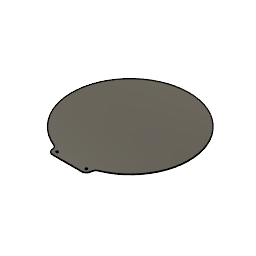
Delta Build Sheet (Autodesk Fusion 360 design; units mm, degrees)
part number: 180mm Square Bed
Autodesk Fusion 360 part; units mm, degrees
sketch "Round Bed" plane through (0, 0, 0) normal (0, 0, 1) x (1, 0, 0)
  line L0 (-90.1561, -90.1561) -> (90.1561, -90.1561) construction
  line L1 (90.1561, -90.1561) -> (90.1561, 90.1561) construction
  line L2 (90.1561, 90.1561) -> (-90.1561, 90.1561) construction
  line L3 (-90.1561, 90.1561) -> (-90.1561, -90.1561) construction
  line L4 (-90.1561, -90.1561) -> (90.1561, 90.1561) construction
  line L5 (90.1561, -90.1561) -> (-90.1561, 90.1561) construction
  line L6 (-31.875, -137.5) -> (31.875, -137.5)
  line L7 (0, 0) -> (0, -137.5) construction
  arc A0 (-42.0024, -127.3726) -> (-31.875, -137.5) centre (-31.875, -127.3726) ccw
  arc A1 (-42.0024, -127.3726) -> (-48.2938, -117.9998) centre (-52.1298, -127.3726) ccw
  arc A2 (31.875, -137.5) -> (42.0024, -127.3726) centre (31.875, -127.3726) ccw
  arc A3 (48.2938, -117.9998) -> (42.0024, -127.3726) centre (52.1298, -127.3726) ccw
  circle A4 centre (-31.875, -127.3726) radius 2
  circle A5 centre (31.875, -127.3726) radius 2
  arc A6 (48.2938, -117.9998) -> (-48.2938, -117.9998) centre (0, 0) ccw
  dimension "d4" = 255
  dimension "d6" = 63.75
  dimension "d7" = 137.5
  dimension "d10" = 4
  constraint coincident L7.start A6.centre
  constraint horizontal L0
  constraint perpendicular L0 L1
  constraint parallel L0 L2
  constraint parallel L1 L3
  constraint coincident L4 L7.start
  constraint coincident L5 L7.start
  constraint coincident L0.start A6
  constraint coincident L0.end A6
  constraint equal L2 L3
  constraint horizontal L6
  constraint midpoint L6 L7.end
  constraint vertical L7
  constraint tangent L6 A0
  constraint tangent A1 A6
  constraint tangent L6 A2
  constraint tangent A3 A6
  constraint tangent A2 A3
  constraint equal A0 A2
  constraint equal A0 A1
  constraint equal A2 A3
  constraint horizontal A2.centre A3.centre
  constraint tangent A0 A1
  constraint concentric A0 A4
  constraint concentric A2 A5
  constraint equal A4 A5
  measures "d4" diameter of A6
  measures "d6" distance of L6.start L6.end
  measures "d7" distance of L7.start L7.end
  measures "d10" diameter of A4
sketch "Square Bed" plane through (0, 0, 0) normal (0, 0, 1) x (1, 0, 0)
  line L0 (-90, -90) -> (90, 90) construction
  line L1 (90, -90) -> (-90, 90) construction
  line L2 (-31.8198, -137.2792) -> (31.8198, -137.2792)
  line L3 (90, -90) -> (90, 90) construction
  arc A0 (48.2308, -117.7871) -> (41.9434, -127.1557) centre (52.0669, -127.1557) ccw
  arc A1 (48.2308, -117.7871) -> (-48.2308, -117.7871) centre (0, 0) ccw
  line L4 (-90, 90) -> (-90, -90) construction
  arc A2 (-41.9434, -127.1557) -> (-48.2308, -117.7871) centre (-52.0669, -127.1557) ccw
  arc A3 (-41.9434, -127.1557) -> (-31.8198, -137.2792) centre (-31.8198, -127.1557) ccw
  line L5 (-90, -90) -> (90, -90) construction
  line L6 (90, 90) -> (-90, 90) construction
  circle A4 centre (-31.8198, -127.1557) radius 2
  arc A5 (31.8198, -137.2792) -> (41.9434, -127.1557) centre (31.8198, -127.1557) ccw
  circle A6 centre (31.8198, -127.1557) radius 2
  line L7 (0, 0) -> (0, -137.2792) construction
  dimension "d14" = 63.6396
  dimension "d16" = 4
  dimension "d17" = 180
  dimension "d18" = 127.2792
  dimension "d20" = 137.2792
  constraint coincident A1.centre L7.start
  constraint horizontal L5
  constraint perpendicular L3 L5
  constraint parallel L5 L6
  constraint parallel L3 L4
  constraint coincident A1.centre L0
  constraint coincident A1.centre L1
  constraint coincident L0.start A1
  constraint coincident L1.start A1
  constraint equal L4 L6
  constraint horizontal L2
  constraint midpoint L7.end L2
  constraint vertical L7
  constraint tangent L2 A3
  constraint tangent A1 A2
  constraint tangent L2 A5
  constraint tangent A0 A1
  constraint tangent A0 A5
  constraint equal A3 A5
  constraint horizontal A5.centre A0.centre
  constraint tangent A2 A3
  constraint concentric A3 A4
  constraint concentric A5 A6
  constraint equal A0 A5
  constraint equal A2 A3
  constraint equal A4 A6
  measures "d14" distance of L2.start L2.end
  measures "d16" diameter of A4
  measures "d17" distance of L0.end L1.end
  measures "d18" radius of A1
  measures "d20" distance of L7.end A1.centre
extrude "Round Bed" [suppressed]
extrude "Square Bed (1)" add sketch "Square Bed" along normal blind 1
equation "d4 = Round_Bed_Size"
equation "d6 = d4 / 4"
equation "d7 = d4 / 2 + 10 mm"
equation "Round_Bed_Size = 255 mm"
equation "Square_Bed_Size = 180 mm"
equation "d14 = ( d18 * 2 ) / 4"
equation "d17 = Square_Bed_Size"
equation "d20 = d18 + 10 mm"
